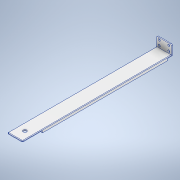
# Autodesk Inventor part: camera_stand
Saved by Autodesk Inventor 2020 (Build 240168000, 168)
## iProperties
Created: 2020-06-26
Part Number: camera_stand
Material: アルミニウム 6061
Document SubType Name: Modeling
Designer: haya
Density: 2.7 g/cm^3
Appearance: アルミニウム - フラット
Author: haya
Autodesk Inventor part; units mm, degrees
ref_plane "YZ Plane" through (0, 0, 0) normal (1, 0, 0) x (0, 1, 0)
ref_plane "XZ Plane" through (0, 0, 0) normal (0, 1, 0) x (-1, 0, 0)
ref_plane "XY Plane" through (0, 0, 0) normal (0, 0, 1) x (1, 0, 0)
sketch "スケッチ1" plane through (0, 0, 0) normal (0, 0, 1) x (1, 0, 0)
  line L0 (0, 0) -> (30, 0)
  line L1 (30, 0) -> (30, 20)
  line L2 (30, 20) -> (0, 20)
  line L3 (0, 20) -> (0, 0)
  dimension "d0" = 30
  dimension "d1" = 20
  constraints: 8 end point, 2 parallel, 1 horizontal, 1 perpendicular
  measures "d0" distance of L0.start L0.end
  measures "d1" distance of L2.end L0.start
extrude "押し出し1" add sketch "スケッチ1" along normal blind 2
sketch "スケッチ2" plane through (0, 0, 2) normal (0, 0, 1) x (1, 0, 0)
  line L0 (0, 20) -> (0, 0) projected
  line L1 (0, 0) -> (30, 0)
  line L2 (30, 0) -> (30, 2)
  line L3 (30, 2) -> (0, 2)
  line L4 (0, 2) -> (0, 0)
  dimension "d4" = 2
  constraints: 8 end point, 2 parallel, 1 coincident, 1 horizontal, 1 perpendicular
  measures "d4" distance between parallel lines of L1 L3
extrude "押し出し2" add sketch "スケッチ2" along normal blind 300
fillet "フィレット1" radius 2 4 edges at (30, 20, 1) (0, 20, 1) (30, 1, 302) (0, 1, 302)
sketch "スケッチ3" plane through (0, 0, 0) normal (0, 0, -1) x (-1, 0, 0)
  line L0 (-28, 20) -> (-2, 20) projected
  line L1 (-15, 20) -> (-15, 0)
  line L2 (-2, 0) -> (-28, 0) projected
  point P0 (0, 0)
  point P1 (-24.7395, 16)
  point P2 (-5.2605, 16)
  point P3 (-24.7395, 6)
  point P4 (-5.2605, 6)
  dimension "d8" = 4
  dimension "d9" = 10
  constraints: 2 end point, 2 midpoint, 2 symmetric about line
  measures "d8" distance from line of point (-24.739, 16) L0
  measures "d9" distance of point (-24.739, 6) point (-24.739, 16)
hole "穴1" at (24.7395, 16, 0) at (5.2605, 16, 0) at (24.7395, 6, 0) at (5.2605, 6, 0) direction (0, 0, 1) diameter 4.5 end through all
sketch "スケッチ4" plane through (0, 2, 2) normal (0, 1, 0) x (1, 0, 0)
  line L0 (2, -300) -> (28, -300) projected
  line L1 (15, -300) -> (15, 2) construction
  line L2 (28, 2) -> (2, 2) projected
  point P0 (0, 2)
  point P1 (15, -280)
  dimension "d17" = 20
  constraints: 2 end point, 2 midpoint, 1 point on line
  measures "d17" distance from line of point (15, -280) L0
hole "穴2" at (15, 2, 282) direction (0, -1, 0) diameter 7 end through all
sketch "スケッチ5" plane through (0, 2, 2) normal (0, 1, 0) x (1, 0, 0)
  line L0 (30, 0) -> (30, -298) projected
  line L1 (28, -8) -> (30, -8)
  line L2 (30, -8) -> (30, -260)
  line L3 (30, -260) -> (28, -260)
  line L4 (28, -260) -> (28, -8)
  line L5 (28, 2) -> (2, 2) projected
  line L6 (28, -300) -> (2, -300) projected
  line L7 (0, 0) -> (30, 0) projected
  line L8 (15, 0) -> (15, -300)
  line L9 (0, 0) -> (0, -298)
  line L10 (2, -8) -> (0, -8)
  line L11 (0, -8) -> (0, -260)
  line L12 (0, -260) -> (2, -260)
  line L13 (2, -260) -> (2, -8)
  point P0 (0, 2)
  dimension "d25" = 10
  dimension "d26" = 2
  dimension "d27" = 40
  constraints: 20 end point, 5 symmetric about line, 2 midpoint, 2 parallel, 2 point on line, 1 horizontal, 1 perpendicular
  measures "d25" distance from line of L1.end L5
  measures "d26" distance between parallel lines of L0 L4
  measures "d27" distance from line of L2.end L6
extrude "押し出し3" add sketch "スケッチ5" against normal blind 6
fillet "フィレット2" radius 1 4 edges at (29.4142, 2, 301.4142) (15, 2, 302) (0.5858, 2, 301.4142) (0, 2, 151)
